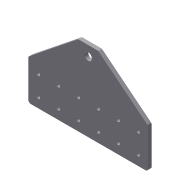
# Autodesk Inventor part: Frame_MidRollerPlate
Saved by Autodesk Inventor 2012 (Build 160160000, 160)
## iProperties
Created: 2012-01-09
Part Number: Frame_MidRollerPlate
Material: Aluminum-6061
Document SubType Name: Modeling
Designer: JesseK
Mass: 154.46 g
Surface Area: 270.226 cm^2
Volume: 56.9965 cm^3
Density: 2.71 g/cm^3
Author: JesseK
Autodesk Inventor part; units mm, degrees
ref_plane "YZ Plane" through (0, 0, 0) normal (1, 0, 0) x (0, 1, 0)
ref_plane "XZ Plane" through (0, 0, 0) normal (0, 1, 0) x (-1, 0, 0)
ref_plane "XY Plane" through (0, 0, 0) normal (0, 0, 1) x (1, 0, 0)
sketch "Sketch1" plane through (0, 0, 0) normal (0, 0, 1) x (1, 0, 0)
  line L0 (0, 0) -> (152.4, 0)
  line L1 (152.4, 0) -> (152.4, 101.6)
  line L2 (152.4, 101.6) -> (0, 101.6)
  line L3 (0, 101.6) -> (0, 0)
  dimension "d0" = 152.4
  dimension "d1" = 101.6
  constraints: 8 end point, 2 parallel, 1 horizontal, 1 perpendicular
  measures "d0" distance of L1.end L2.end
  measures "d1" distance of L0.end L1.end
extrude "Extrusion1" add sketch "Sketch1" along normal blind 4.7625
sketch "Sketch2" plane through (0, 0, 4.7625) normal (0, 0, 1) x (1, 0, 0)
  line L0 (0, 0) -> (0, 101.6) projected
  line L1 (0, 101.6) -> (152.4, 101.6) projected
  circle A0 centre (76.2, 88.9) radius 4.7625
  dimension "d4" = 76.2
  dimension "d5" = 12.7
  dimension "d25" = 9.525
  constraints: 1 centre point
  measures "d4" distance from line of L0 A0.centre
  measures "d5" distance from line of L1 A0.centre
  measures "d25" diameter of A0
extrude "Extrusion2" cut sketch "Sketch2" against normal up to next
sketch "Sketch3" plane through (0, 0, 4.7625) normal (0, 0, 1) x (1, 0, 0)
  line L0 (0, 0) -> (0, 101.6) projected
  line L1 (152.4, 0) -> (0, 0) projected
  circle A0 centre (12.7, 12.7) radius 2.3813
  dimension "d8" = 4.7625
  dimension "d9" = 12.7
  dimension "d10" = 12.7
  constraints: 1 centre point
  measures "d8" diameter of A0
  measures "d9" distance from line of L1 A0.centre
  measures "d10" distance from line of L0 A0.centre
extrude "Extrusion3" cut sketch "Sketch3" against normal up to next
pattern_linear "Rectangular Pattern1" count 6 spacing 25.4 along (1, 0, 0) count 2 spacing 25.4 along (0, 1, 0) of "Extrusion3"
sketch "Sketch4" plane through (0, 0, 4.7625) normal (0, 0, 1) x (1, 0, 0)
  line L0 (0, 0) -> (0, 101.6) projected
  line L1 (152.4, 101.6) -> (152.4, 0) projected
  line L2 (0, 101.6) -> (152.4, 101.6) projected
  line L3 (0, 50.8) -> (63.5, 101.6)
  line L4 (0, 101.6) -> (0, 50.8)
  line L5 (63.5, 101.6) -> (0, 101.6)
  line L6 (152.4, 101.6) -> (152.4, 50.8)
  line L7 (88.9, 101.6) -> (152.4, 50.8)
  line L8 (152.4, 101.6) -> (88.9, 101.6)
  dimension "d19" = 63.5
  dimension "d20" = 63.5
  dimension "d21" = 50.8
  constraints: 12 end point, 2 collinear, 2 midpoint, 2 point on line, 1 parallel, 1 perpendicular
  measures "d19" distance of L3.end L0.end
  measures "d20" distance of L1.start L7.start
  measures "d21" distance of L0.start L3.start
extrude "Extrusion4" cut sketch "Sketch4" against normal up to next
fillet "Fillet1" radius 3.175 6 edges at (63.5, 101.6, 2.3813) (88.9, 101.6, 2.3813) (152.4, 50.8, 2.3813) (152.4, 0, 2.3813) (0, 0, 2.3813) (0, 50.8, 2.3813)
body "Solid1"
